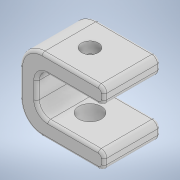
# Autodesk Inventor part: Cable-Holder
Saved by Autodesk Inventor 2021 (Build 250183000, 183)
## iProperties
Created: 2021-09-04
Part Number: Cable-Holder
Material: Genérico
Document SubType Name: Modeling
Designer: Diego.labarca
Density: 1 g/cm^3
Appearance: Valor por defecto
Author: Diego.labarca
Autodesk Inventor part; units mm, degrees
ref_plane "YZ Plane" through (0, 0, 0) normal (1, 0, 0) x (0, 1, 0)
ref_plane "XZ Plane" through (0, 0, 0) normal (0, 1, 0) x (-1, 0, 0)
ref_plane "XY Plane" through (0, 0, 0) normal (0, 0, 1) x (1, 0, 0)
sketch "Boceto1" plane through (0, 0, 0) normal (0, 1, 0) x (1, 0, 0)
  line L0 (-7.5, 5) -> (7.5, 5)
  line L1 (7.5, 5) -> (7.5, -5)
  line L2 (7.5, -5) -> (-7.5, -5)
  line L3 (-7.5, -5) -> (-7.5, 5)
  line L4 (-10.5, 0) -> (10.5, 0) projected
  line L5 (0, -7) -> (0, 7) projected
  dimension "d0" = 15
  dimension "d1" = 10
  constraints: 8 end point, 2 parallel, 1 horizontal, 1 perpendicular, 2 other
  measures "d0" distance of L1.end L2.end
  measures "d1" distance of L0.end L1.end
extrude "Extrusión1" add sketch "Boceto1" along normal blind 3
sketch "Boceto2" plane through (-7.5, 0, 5) normal (0, 0, 1) x (1, 0, 0)
  line L0 (15, 3) -> (0, 3) projected
  line L1 (0, 3) -> (0, 13)
  line L2 (0, 13) -> (15, 13)
  line L3 (15, 13) -> (15, 10)
  line L4 (15, 10) -> (3, 10)
  line L5 (3, 10) -> (3, 3)
  point P0 (7.5, 0)
  dimension "d5" = 10
  dimension "d6" = 3
  dimension "d7" = 15
  dimension "d8" = 12
  constraints: 10 end point, 3 perpendicular, 2 vertical, 1 point on line
  measures "d5" distance of L0.end L1.end
  measures "d6" distance of L2.end L3.end
  measures "d7" distance of L1.end L2.end
  measures "d8" distance of L3.end L4.end
extrude "Extrusión2" add sketch "Boceto2" against normal up to surface (10 mm away)
sketch "Boceto3" plane through (-7.5, 13, 5) normal (0, 1, 0) x (1, 0, 0)
  circle A0 centre (7.5, 5) radius 1.5
  dimension "d11" = 3
  constraints: 1 centre point, 1 coincident
  measures "d11" diameter of A0
extrude "Extrusión3" cut sketch "Boceto3" against normal up to surface (3 mm away)
fillet "Empalme1" radius 2 2 edges at (-4.5, 10, 0) (-4.5, 3, 0)
sketch "Boceto4" plane through (0, 0, 0) normal (0, -1, 0) x (-1, 0, 0)
  circle A0 centre (0, 0) radius 2
  dimension "d15" = 4
  constraints: 1 centre point, 1 coincident
  measures "d15" diameter of A0
extrude "Extrusión4" cut sketch "Boceto4" against normal up to surface (3 mm away)
fillet "Empalme2" radius 1 4 edges at (7.5, 0, 0) (7.5, 3, 0) (7.5, 13, 0) (7.5, 10, 0)
fillet "Empalme3" radius 4 2 edges at (-7.5, 13, 0) (-7.5, 0, 0)
fillet "Empalme4" radius 0.5 32 edges at (-6.3284, 1.1716, -5) (-7.5, 6.5, -5) (-6.3284, 11.8284, -5) (1.5, 13, -5) (7.2071, 12.7071, -5) (7.5, 11.5, -5) (7.2071, 10.2929, -5) (2, 10, -5) (-3.9142, 9.4142, -5) (-4.5, 6.5, -5) (-3.9142, 3.5858, -5) (2, 3, -5) (7.2071, 2.7071, -5) (7.5, 1.5, -5) (7.2071, 0.2929, -5) (1.5, 0, -5) (7.2071, 0.2929, 5) (7.5, 1.5, 5) (7.2071, 2.7071, 5) (2, 3, 5) (-3.9142, 3.5858, 5) (-4.5, 6.5, 5) (-3.9142, 9.4142, 5) (2, 10, 5) (7.2071, 10.2929, 5) (7.5, 11.5, 5) (7.2071, 12.7071, 5) (1.5, 13, 5) (-6.3284, 11.8284, 5) (-7.5, 6.5, 5) (-6.3284, 1.1716, 5) (1.5, 0, 5)
chamfer "Chaflán1" distance 1 angle 45 1 edges at (-1.5, 10, 0)
